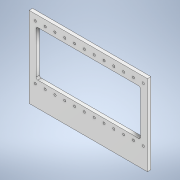
# Autodesk Inventor part: Center Wall
Saved by Autodesk Inventor 2021 (Build 250183000, 183)
## iProperties
Created: 2022-07-24
Part Number: Center Wall
Material: ABS Plastic
Document SubType Name: Modeling
Designer: erics
Mass: 224.843 g
Surface Area: 816.547 cm^2
Volume: 212.116 cm^3
Density: 1.06 g/cm^3
Appearance: Smooth - White
Author: erics
Autodesk Inventor part; units mm, degrees
ref_plane "YZ Plane" through (0, 0, 0) normal (1, 0, 0) x (0, 1, 0)
ref_plane "XZ Plane" through (0, 0, 0) normal (0, 1, 0) x (-1, 0, 0)
ref_plane "XY Plane" through (0, 0, 0) normal (0, 0, 1) x (1, 0, 0)
sketch "Sketch1" plane through (0, 0, 0) normal (0, 0, 1) x (1, 0, 0)
  line L0 (0, 0) -> (214.63, 0)
  line L1 (214.63, 0) -> (214.63, 146.05)
  line L2 (214.63, 146.05) -> (0, 146.05)
  line L3 (0, 146.05) -> (0, 0)
  line L4 (0, 146.05) -> (-6.35, 146.05) construction
  line L5 (-6.35, 146.05) -> (-6.35, 0) construction
  line L6 (-6.35, 0) -> (0, 0) construction
  line L7 (214.63, 0) -> (220.98, 0) construction
  line L8 (220.98, 0) -> (220.98, 146.05) construction
  line L9 (214.63, 146.05) -> (220.98, 146.05) construction
  line L10 (-8.255, 0) -> (-8.255, 93.2539)
  line L11 (222.885, 0) -> (222.885, 86.8023)
  line L12 (-8.255, 0) -> (222.885, 0)
  point P0 (-3.175, 146.05)
  point P1 (217.805, 146.05)
  point P2 (107.315, 0)
  dimension "d0" = 146.05
  dimension "d1" = 214.63
  dimension "d17" = 6.35
  dimension "d18" = 6.35
  dimension "d19" = 227.33
  dimension "d21" = 220.98
  dimension "d56" = 5.08
  dimension "d57" = 231.14
  constraints: 26 end point, 5 horizontal, 4 midpoint, 4 perpendicular, 2 parallel, 2 vertical, 1 horizontal alignment
  measures "d0" distance of L2.end L0.start
  measures "d1" distance of L1.end L2.end
  measures "d17" distance between parallel lines of L3 L5
  measures "d18" distance between parallel lines of L1 L8
  measures "d19" distance between parallel lines of L8 L5
  measures "d21" distance of point (217.805, 146.05) point (-3.175, 146.05)
  measures "d56" distance from line of point (-3.175, 146.05) L10
  measures "d57" distance between parallel lines of L11 L10
extrude "Extrusion1" add sketch "Sketch1" along normal mid plane 6.35
sketch "Sketch2" plane through (0, 0, 3.175) normal (0, 0, 1) x (1, 0, 0)
  circle A0 centre (11.5378, 135.236) radius 2
  circle A1 centre (11.5378, 36.736) radius 2
  line L0 (6.6378, 141.986) -> (16.4378, 141.986) construction
  line L1 (16.4378, 141.986) -> (16.4378, 29.986) construction
  line L2 (16.4378, 29.986) -> (6.6378, 29.986) construction
  line L3 (6.6378, 29.986) -> (6.6378, 141.986) construction
  line L4 (11.5378, 36.736) -> (11.5378, 135.236) construction
  line L5 (0, 0) -> (214.63, 0) construction
  line L6 (0, 146.05) -> (0, 0) projected
  line L7 (-6.35, 146.05) -> (-6.35, 0) construction
  line L8 (6.6378, 128.336) -> (8.2378, 128.336) construction
  line L9 (8.2378, 128.336) -> (8.2378, 43.636) construction
  line L10 (8.2378, 43.636) -> (6.6378, 43.636) construction
  line L11 (6.6378, 43.636) -> (6.6378, 128.336) construction
  line L12 (16.4378, 128.336) -> (14.8378, 128.336) construction
  line L13 (14.8378, 128.336) -> (14.8378, 43.636) construction
  line L14 (14.8378, 43.636) -> (16.4378, 43.636) construction
  line L15 (16.4378, 43.636) -> (16.4378, 128.336) construction
  line L16 (214.63, 146.05) -> (0, 146.05) projected
  line L17 (-8.255, 0) -> (-8.255, 93.2539) projected
  point P0 (11.5378, 141.986)
  point P1 (11.5378, 85.986)
  point P2 (16.4378, 85.986)
  point P3 (14.8378, 85.986)
  point P4 (8.2378, 85.986)
  dimension "d4" = 98.5
  dimension "d5" = 4
  dimension "d7" = 9.8
  dimension "d8" = 141.986
  dimension "d22" = 112
  dimension "d23" = 6.6
  dimension "d24" = 13.65
  dimension "d58" = 19.7928
  constraints: 26 end point, 7 parallel, 5 midpoint, 3 horizontal, 3 horizontal alignment, 3 perpendicular, 2 centre point, 2 equal length, 2 point on line, 2 vertical alignment, 1 equal radius
  measures "d4" distance of L4.start L4.end
  measures "d5" diameter of A0
  measures "d7" distance of L0.start L0.end
  measures "d8" distance between parallel lines of L5 L0
  measures "d22" distance of L0.end L1.end
  measures "d23" distance between parallel lines of L13 L9
  measures "d24" distance between parallel lines of L0 L12
  measures "d58" distance between parallel lines of L4 L17
extrude "Extrusion2" cut sketch "Sketch2" against normal blind 9.525
pattern_linear "Rectangular Pattern1" count 12 spacing 17.78 along (1, 0, 0) of "Extrusion2"
sketch "Sketch3" plane through (0, 0, 3.175) normal (0, 0, 1) x (1, 0, 0)
  line L0 (12.7, 44.45) -> (201.93, 44.45)
  line L1 (201.93, 44.45) -> (201.93, 127)
  line L2 (201.93, 127) -> (12.7, 127)
  line L3 (12.7, 127) -> (12.7, 44.45)
  line L4 (214.63, 0) -> (214.63, 146.05) projected
  line L5 (0, 146.05) -> (0, 0) projected
  line L6 (214.63, 146.05) -> (0, 146.05) projected
  line L7 (0, 0) -> (214.63, 0) projected
  dimension "d49" = 12.7
  dimension "d50" = 12.7
  dimension "d51" = 19.05
  dimension "d52" = 44.45
  constraints: 8 end point, 2 parallel, 1 horizontal, 1 perpendicular
  measures "d49" distance between parallel lines of L4 L1
  measures "d50" distance between parallel lines of L5 L3
  measures "d51" distance between parallel lines of L6 L2
  measures "d52" distance between parallel lines of L7 L0
extrude "Extrusion3" cut sketch "Sketch3" against normal through all contours L3 L2 L1 L0
fillet "Fillet1" radius 3.175 4 edges at (12.7, 44.45, 0) (12.7, 127, 0) (201.93, 44.45, 0) (201.93, 127, 0)
sketch "Sketch5" plane through (0, 0, 3.175) normal (0, -1, 0) x (1, 0, 0)
  line L0 (0, -6.35) -> (0, 0) projected
  point P0 (0, -3.175)
  point P1 (67.945, -3.175)
  point P2 (0, -3.175)
  point P3 (-8.255, -3.175)
  point P4 (-8.255, -3.175)
  point P5 (-8.255, -3.175)
  point P6 (139.065, -3.175)
  point P7 (0, -3.175)
  dimension "d69" = 76.2
  dimension "d70" = 147.32
  constraints: 2 horizontal alignment, 2 midpoint
  measures "d69" distance of point (67.945, -3.175) point (-8.255, -3.175)
  measures "d70" distance of point (-8.255, -3.175) point (139.065, -3.175)
hole "Hole1" at (67.945, 0, 0) at (139.065, 0, 0) direction (0, 1, 0) diameter 3.9688 depth 9.525 tip angle 118
equation "\"d18\" = d17"
body "Solid1"
